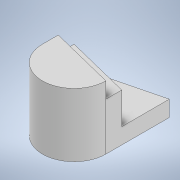
# Autodesk Inventor part: 零件6
Saved by Autodesk Inventor 2020 (Build 240168000, 168)
## iProperties
Created: 2020-09-19
Part Number: 零件6
Material: 一般
Document SubType Name: Modeling
Designer: User
Density: 1 g/cm^3
Appearance: 預設
Mass: 55.1327 g
Surface Area: 101.068 cm^2
Volume: 55.1327 cm^3
Author: User
Autodesk Inventor part; units mm, degrees
ref_plane "YZ Plane" through (0, 0, 0) normal (1, 0, 0) x (0, 1, 0)
ref_plane "XZ Plane" through (0, 0, 0) normal (0, 1, 0) x (-1, 0, 0)
ref_plane "XY Plane" through (0, 0, 0) normal (0, 0, 1) x (1, 0, 0)
sketch "草圖1" plane through (0, 0, 0) normal (0, 1, 0) x (-1, 0, 0)
  line L0 (-20, 0) -> (-20, -40)
  line L1 (20, -30) -> (20, 0)
  line L2 (-20, 0) -> (20, -10)
  line L3 (-20, -10) -> (20, -20)
  arc A0 (20, 0) -> (-20, 0) centre (0, 0) ccw
  line L4 (-20, -40) -> (20, -30)
  dimension "d11" = 20
  dimension "d13" = 10
  dimension "d14" = 20
  dimension "d16" = 40
  dimension "d17" = 30
  dimension "d18" = 40
  dimension "d19" = 30
  constraints: 10 end point, 3 point on line, 2 parallel, 2 point on circle, 1 centre point, 1 coincident
  measures "d11" radius of A0
  measures "d13" distance of L2.end L1.end
  measures "d14" distance of L3.end L1.end
  measures "d16" distance between parallel lines of L0 L1
  measures "d17" distance of L1.start L1.end
  measures "d18" vertical distance of A0.centre L0.end
  measures "d19" distance of L0.end L3.start
extrude "擠出1" add sketch "草圖1" along normal blind 40 contours A0 L1 L2
extrude "擠出2" add sketch "草圖1" along normal blind 30 contours L2 L1 L3 L0
extrude "擠出3" add sketch "草圖1" along normal blind 10
